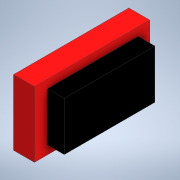
# Autodesk Inventor part: Periph_Screen
Saved by Autodesk Inventor 2020 (Build 240168000, 168)
## iProperties
Created: 2022-01-28
Part Number: Periph_Screen
Material: Generic
Document SubType Name: Modeling
Designer: danie
Density: 1 g/cm^3
Appearance: Default
Author: danie
Autodesk Inventor part; units mm, degrees
ref_plane "YZ Plane" through (0, 0, 0) normal (1, 0, 0) x (0, 1, 0)
ref_plane "XZ Plane" through (0, 0, 0) normal (0, 1, 0) x (-1, 0, 0)
ref_plane "XY Plane" through (0, 0, 0) normal (0, 0, 1) x (1, 0, 0)
sketch "Sketch1" plane through (0, 0, 0) normal (1, 0, 0) x (0, 1, 0)
  line L0 (0, 0) -> (-39.878, 0)
  line L1 (-39.878, 0) -> (-39.878, -70.104)
  line L2 (-39.878, -70.104) -> (0, -70.104)
  line L3 (0, -70.104) -> (0, 0)
  dimension "d0" = 39.878
  dimension "d1" = 70.104
  constraints: 8 end point, 2 parallel, 1 horizontal, 1 perpendicular
  measures "d0" distance of L2.end L1.end
  measures "d1" distance of L1.end L0.end
extrude "Extrusion1" add sketch "Sketch1" along normal blind 12.7
sketch "Sketch2" plane through (12.7, 0, 0) normal (1, 0, 0) x (0, 0, -1)
  line L0 (7.9684, 0) -> (7.9684, -5.08) construction
  line L1 (34.6892, -39.7724) -> (34.6892, -34.6924) construction
  line L2 (34.6892, -39.7724) -> (39.7692, -39.7724) construction
  line L3 (7.9684, -5.08) -> (63.0635, -5.08)
  line L4 (63.0635, -5.08) -> (63.0635, -34.6924)
  line L5 (63.0635, -34.6924) -> (7.9684, -34.6924)
  line L6 (7.9684, -34.6924) -> (7.9684, -5.08)
  point P0 (0, 0)
  dimension "d4" = 5.08
  dimension "d5" = 5.08
  dimension "d6" = 90
  constraints: 14 end point, 2 horizontal, 2 parallel, 2 perpendicular, 2 vertical
  measures "d4" distance of L0.start L0.end
  measures "d5" distance of L1.start L1.end
  measures "d6" angle of L2 L1
extrude "Extrusion2" add sketch "Sketch2" along normal blind 10.16
body "Solid1"
